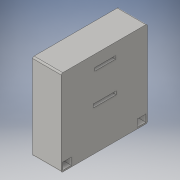
# Autodesk Inventor part: frame_front
Saved by Autodesk Inventor 2016 (Build 200138000, 138)
## iProperties
Created: 2017-09-22
Part Number: frame_front
Material: Generic
Document SubType Name: Modeling
Designer: Student
Density: 1 g/cm^3
Appearance: Default
Author: Student
Autodesk Inventor part; units mm, degrees
ref_plane "YZ Plane" through (0, 0, 0) normal (1, 0, 0) x (0, 1, 0)
ref_plane "XZ Plane" through (0, 0, 0) normal (0, 1, 0) x (-1, 0, 0)
ref_plane "XY Plane" through (0, 0, 0) normal (0, 0, 1) x (1, 0, 0)
sketch "Sketch1" plane through (0, 0, 0) normal (1, 0, 0) x (0, 1, 0)
  line L0 (7.62, 0) -> (74.93, 0)
  line L1 (76.2, -1.27) -> (76.2, -74.93)
  line L2 (74.93, -76.2) -> (7.62, -76.2)
  line L3 (7.62, -7.62) -> (7.62, -1.27)
  line L4 (7.62, -68.58) -> (7.62, -74.93)
  line L5 (38.5844, -48.4886) -> (35.5872, -48.4886)
  line L6 (35.5872, -48.4886) -> (35.5872, -28.2956)
  line L7 (35.5872, -28.2956) -> (38.5844, -28.2956)
  line L8 (38.5844, -28.2956) -> (38.5844, -48.4886)
  line L9 (1.27, -8.89) -> (7.62, -8.89)
  line L10 (7.62, -7.62) -> (7.62, -8.89)
  line L11 (1.27, -67.31) -> (7.62, -67.31)
  line L12 (7.62, -67.31) -> (7.62, -68.58)
  line L13 (0, -8.89) -> (0, -67.31)
  line L14 (7.62, 0) -> (1.27, 0)
  line L15 (0, -1.27) -> (0, -8.89)
  line L16 (0, 0) -> (1.27, 0)
  line L17 (7.62, -1.27) -> (1.27, -1.27)
  line L18 (1.27, -1.27) -> (1.27, -8.89)
  line L19 (7.62, -76.2) -> (1.27, -76.2)
  line L20 (0, -74.93) -> (0, -67.31)
  line L21 (0, -76.2) -> (1.27, -76.2)
  line L22 (7.62, -74.93) -> (1.27, -74.93)
  line L23 (1.27, -74.93) -> (1.27, -67.31)
  line L24 (63.1716, -29.6545) -> (65.8894, -29.6545)
  arc A0 (76.2, -1.27) -> (74.93, 0) centre (74.93, -1.27) ccw
  arc A1 (74.93, -76.2) -> (76.2, -74.93) centre (74.93, -74.93) ccw
  arc A2 (1.27, 0) -> (0, -1.27) centre (1.27, -1.27) ccw
  arc A3 (0, -74.93) -> (1.27, -76.2) centre (1.27, -74.93) ccw
  line L25 (63.1716, -29.6545) -> (63.1716, -47.9425)
  line L26 (65.8894, -29.6545) -> (65.8894, -47.9425)
  line L27 (65.8894, -47.9425) -> (63.1716, -47.9425)
  dimension "d8" = 12.7
  dimension "d11" = 25.4
  dimension "d18" = 10.6045
  dimension "d39" = 2.9972
  dimension "d40" = 20.193
  dimension "d44" = 1.27
  dimension "d50" = 2.7178
  dimension "d51" = 1.27
  dimension "d52" = 1.27
  dimension "d53" = 1.27
  dimension "d54" = 1.27
  dimension "d55" = 18.288
  constraints: 56 end point, 11 perpendicular, 8 point on circle, 8 point on line, 8 tangent, 7 horizontal, 5 vertical, 4 centre point, 1 parallel
  measures "d39" distance of L5.start L5.end
  measures "d40" distance of L5.end L6.end
  measures "d44" distance of L16.start L16.end
  measures "d50" distance of L24.start L24.end
  measures "d51" radius of A0
  measures "d52" radius of A1
  measures "d53" radius of A2
  measures "d54" radius of A3
  measures "d55" distance of L24.start L25.end
extrude "Extrusion3" add sketch "Sketch1" along normal blind 25.4
body "Solid3"
